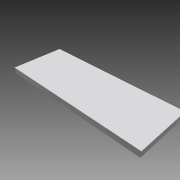
# Autodesk Inventor part: YagiPSUSide
Saved by Autodesk Inventor 2014 (Build 180170000, 170)
## iProperties
Created: 2015-05-23
Part Number: YagiPSUSide
Material: Generic
Document SubType Name: Modeling
Designer: Owner
Density: 1 g/cm^3
Appearance: Aluminum - Polished
Author: Owner
Autodesk Inventor part; units mm, degrees
ref_plane "YZ Plane" through (0, 0, 0) normal (1, 0, 0) x (0, 1, 0)
ref_plane "XZ Plane" through (0, 0, 0) normal (0, 1, 0) x (-1, 0, 0)
ref_plane "XY Plane" through (0, 0, 0) normal (0, 0, 1) x (1, 0, 0)
sketch "Sketch1" plane through (0, 0, 0) normal (0, 1, 0) x (-1, 0, 0)
  line L0 (-73.8377, 26.349) -> (78.5623, 26.349)
  line L1 (78.5623, 26.349) -> (78.5623, -30.801)
  line L2 (78.5623, -30.801) -> (-73.8377, -30.801)
  line L3 (-73.8377, -30.801) -> (-73.8377, 26.349)
  point P0 (0, 0)
  dimension "d0" = 152.4
  dimension "d1" = 57.15
  constraints: 8 end point, 2 parallel, 1 horizontal, 1 perpendicular
  measures "d0" distance of L0.start L0.end
  measures "d1" distance of L0.end L1.end
extrude "Extrusion1" add sketch "Sketch1" along normal blind 6.35
sketch "Sketch2" plane through (73.8377, 0, 26.349) normal (1, 0, 0) x (0, 0, -1)
  point P0 (49.53, 3.175)
hole "Hole1" at (73.8377, 3.175, -23.181) direction (-1, 0, 0) diameter 1.1811 depth 2.286 tip angle 120 thread size "0-80 UNF" class "2B" standard "ANSI Unified Screw Threads"
sketch "Sketch3" plane through (-78.5623, 0, -30.801) normal (-1, 0, 0) x (0, 0, 1)
  point P0 (7.62, 3.175)
hole "Hole3" at (-78.5623, 3.175, -23.181) direction (1, 0, 0) diameter 1.1811 depth 2.286 tip angle 120 thread size "0-80 UNF" class "2B" standard "ANSI Unified Screw Threads"
sketch "Sketch4" plane through (-78.5623, 0, 26.349) normal (0, 0, 1) x (1, 0, 0)
  point P0 (6.35, 3.175)
hole "Hole5" at (-72.2123, 3.175, 26.349) direction (0, 0, -1) diameter 1.778 depth 57.15
pattern_linear "Rectangular Pattern1" count 4 spacing 12.7 along (0, 0, 1) of "Hole3"
pattern_linear "Rectangular Pattern2" count 4 spacing 12.7 along (0, 0, 1) of "Hole1"
pattern_linear "Rectangular Pattern3" count 12 spacing 12.7 along (1, 0, 0) of "Hole5"
sketch "Sketch5" plane through (0, 6.35, 0) normal (0, 1, 0) x (1, 0, 0)
  point P0 (18.6377, 23.826)
hole "Hole7" at (18.6377, 6.35, -23.826) direction (0, -1, 0) diameter 3.4544 depth 6.35
pattern_linear "Rectangular Pattern4" count 2 spacing 12.7 along (-1, 0, 0) of "Hole7"
sketch "Sketch6" plane through (0, 6.35, 0) normal (0, 1, 0) x (1, 0, 0)
  point P0 (59.4877, 23.5381)
hole "Hole9" at (59.4877, 6.35, -23.5381) direction (0, -1, 0) diameter 1.778 depth 6.35
sketch "Sketch7" plane through (0, 6.35, 0) normal (0, 1, 0) x (1, 0, 0)
  point P0 (42.7237, 23.5381)
hole "Hole11" at (42.7237, 6.35, -23.5381) direction (0, -1, 0) diameter 1.778 depth 6.35
sketch "Sketch8" plane through (0, 6.35, 0) normal (0, 1, 0) x (1, 0, 0)
  point P0 (59.4877, -17.3559)
hole "Hole13" at (59.4877, 6.35, 17.3559) direction (0, -1, 0) diameter 1.778 depth 6.35
sketch "Sketch9" plane through (0, 6.35, 0) normal (0, 1, 0) x (1, 0, 0)
  point P0 (42.7237, -17.3559)
hole "Hole15" at (42.7237, 6.35, 17.3559) direction (0, -1, 0) diameter 1.778 depth 6.35
sketch "Sketch10" plane through (0, 6.35, 0) normal (0, 1, 0) x (1, 0, 0)
  point P0 (33.1987, 10.9651)
hole "Hole17" at (33.1987, 6.35, -10.9651) direction (0, -1, 0) diameter 1.778 depth 6.35
sketch "Sketch11" plane through (0, 6.35, 0) normal (0, 1, 0) x (1, 0, 0)
  point P0 (-41.0963, -8.7834)
hole "Hole19" at (-41.0963, 6.35, 8.7834) direction (0, -1, 0) diameter 1.778 depth 6.35
body "Solid1"
